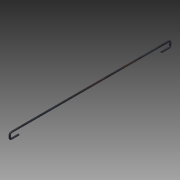
# Autodesk Inventor part: Rudder_Link
Saved by Autodesk Inventor 2011 SP1 (Build 150282100, 282)
## iProperties
Created: 2011-06-11
Part Number: Rudder_Link
Document SubType Name: Modeling
Designer: Andrew G. Meyer
Mass: 0.150374 g
Surface Area: 5.06089 cm^2
Volume: 0.150374 cm^3
Density: 1 g/cm^3
Author: Andrew G. Meyer
Autodesk Inventor part; units mm, degrees
ref_plane "YZ Plane" through (0, 0, 0) normal (1, 0, 0) x (0, 1, 0)
ref_plane "XZ Plane" through (0, 0, 0) normal (0, 1, 0) x (-1, 0, 0)
ref_plane "XY Plane" through (0, 0, 0) normal (0, 0, 1) x (1, 0, 0)
sketch "Sketch1" plane through (0, 0, 0) normal (0, 0, 1) x (1, 0, 0)
  circle A0 centre (0, 0) radius 0.5969
  dimension "d0" = 1.1938
  constraints: 1 centre point, 1 coincident
  measures "d0" diameter of A0
sketch "Sketch2" plane through (0, 0, 0) normal (1, 0, 0) x (0, 1, 0)
  line L0 (0, 0) -> (0, 5.08)
  line L1 (1.27, 6.35) -> (2.8575, 6.35)
  line L2 (4.1275, 5.08) -> (4.1275, -107.95)
  line L3 (0, -107.95) -> (0, -102.87)
  line L4 (2.8575, -109.22) -> (1.27, -109.22)
  arc A0 (4.1275, 5.08) -> (2.8575, 6.35) centre (2.8575, 5.08) ccw
  arc A1 (2.8575, -109.22) -> (4.1275, -107.95) centre (2.8575, -107.95) ccw
  arc A2 (0, -107.95) -> (1.27, -109.22) centre (1.27, -107.95) ccw
  arc A3 (1.27, 6.35) -> (0, 5.08) centre (1.27, 5.08) ccw
  dimension "d1" = 1.27
  dimension "d5" = 1.5875
  dimension "d7" = 115.57
  dimension "d8" = 6.35
  constraints: 10 end point, 8 point on circle, 8 tangent, 4 centre point, 3 equal radius, 2 equal length, 2 parallel, 2 perpendicular, 1 vertical
  measures "d1" radius of A0
  measures "d5" distance of L1.start L1.end
  measures "d7" distance between parallel lines of L4 L1
  measures "d8" distance from line of L1 L0.start
sweep "Sweep1" add profiles "Sketch1" path "Sketch2"
body "Solid1"
